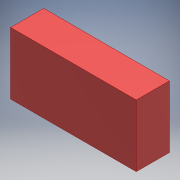
# Autodesk Inventor part: bateria
Saved by Autodesk Inventor 2018 (Build 220112000, 112)
## iProperties
Created: 2018-03-07
Part Number: bateria
Material: Genérico
Document SubType Name: Modeling
Designer: ivanb
Density: 1 g/cm^3
Appearance: Valor por defecto
Author: ivanb
Autodesk Inventor part; units mm, degrees
ref_plane "YZ Plane" through (0, 0, 0) normal (1, 0, 0) x (0, 1, 0)
ref_plane "XZ Plane" through (0, 0, 0) normal (0, 1, 0) x (-1, 0, 0)
ref_plane "XY Plane" through (0, 0, 0) normal (0, 0, 1) x (1, 0, 0)
sketch "Boceto1" plane through (0, 0, 0) normal (0, 1, 0) x (-1, 0, 0)
  line L0 (46.229, 23.8395) -> (-48.771, 23.8395)
  line L1 (-48.771, 23.8395) -> (-48.771, -23.1605)
  line L2 (-48.771, -23.1605) -> (46.229, -23.1605)
  line L3 (46.229, -23.1605) -> (46.229, 23.8395)
  point P0 (0, 0)
  dimension "d0" = 95
  dimension "d1" = 47
  constraints: 8 end point, 2 parallel, 1 horizontal, 1 perpendicular
  measures "d0" distance of L2.end L1.end
  measures "d1" distance of L1.end L0.end
extrude "Extrusión1" add sketch "Boceto1" along normal blind 25
